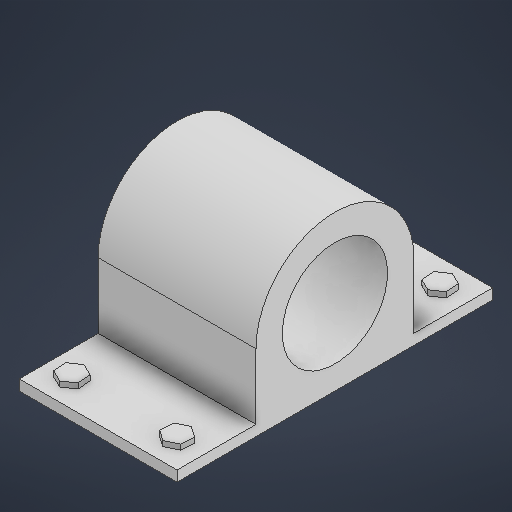
# Autodesk Inventor part: hold down pin
Saved by Autodesk Inventor 2026.1 (Build 301233020, 233B)
## iProperties
Created: 2025-12-30
Part Number: hold down pin
Material: Generic
Document SubType Name: Modeling
Designer: Austin Ngobeni
Density: 1 g/cm^3
Appearance: Default
Author: Austin Ngobeni
Autodesk Inventor part; units mm, degrees
ref_plane "YZ Plane" through (0, 0, 0) normal (1, 0, 0) x (0, 1, 0)
ref_plane "XZ Plane" through (0, 0, 0) normal (0, 1, 0) x (-1, 0, 0)
ref_plane "XY Plane" through (0, 0, 0) normal (0, 0, 1) x (1, 0, 0)
sketch "Sketch1" plane through (0, 0, 0) normal (1, 0, 0) x (0, 1, 0)
  line L0 (-1, 30) -> (1, 30)
  line L1 (1, -30) -> (-1, -30)
  line L2 (-1, -30) -> (-1, 30)
  arc A0 (13.4551, -15) -> (13.4551, 15) centre (13.4551, 0) ccw
  circle A1 centre (13.4551, 0) radius 10
  line L3 (13.4551, 15) -> (1, 15)
  line L4 (13.4551, -15) -> (1, -15)
  line L5 (1, 30) -> (1, 15)
  line L6 (1, -15) -> (1, -30)
  point P0 (0, 0)
  point P1 (0, 30)
  point P2 (1, 0)
  dimension "d0" = 2
  dimension "d1" = 60
  dimension "d2" = 30
  dimension "d3" = 20
  constraints: 14 end point, 4 perpendicular, 3 parallel, 2 centre point, 2 horizontal, 2 point on circle, 2 tangent, 1 coincident, 1 horizontal alignment, 1 midpoint, 1 vertical alignment
  measures "d0" distance of L0.start L0.end
  measures "d1" distance of L0.end L1.start
  measures "d2" diameter of A0
  measures "d3" diameter of A1
extrude "Extrusion1" add sketch "Sketch1" along normal blind 30
sketch "Sketch2" plane through (0, 1, 30) normal (0, 1, 0) x (1, 0, 0)
  circle A0 centre (5, 5) radius 2.5 construction
  line L0 (0, 0) -> (30, 0) projected
  line L1 (15, 0) -> (15, 91.9575) construction
  line L2 (56.6517, 30) -> (-26.6517, 30) construction
  line L3 (0, 0) -> (0, 60) projected
  line L4 (7.0666, 6.4068) -> (7.2516, 3.9137)
  line L5 (7.2516, 3.9137) -> (5.185, 2.5069)
  line L6 (5.185, 2.5069) -> (2.9334, 3.5932)
  line L7 (2.9334, 3.5932) -> (2.7484, 6.0863)
  line L8 (2.7484, 6.0863) -> (4.815, 7.4931)
  line L9 (4.815, 7.4931) -> (7.0666, 6.4068)
  line L10 (22.9334, 6.4068) -> (22.7484, 3.9137)
  line L11 (22.7484, 3.9137) -> (24.815, 2.5069)
  line L12 (24.815, 2.5069) -> (27.0666, 3.5932)
  line L13 (27.0666, 3.5932) -> (27.2516, 6.0863)
  line L14 (27.2516, 6.0863) -> (25.185, 7.4931)
  line L15 (25.185, 7.4931) -> (22.9334, 6.4068)
  line L16 (7.0666, 53.5932) -> (7.2516, 56.0863)
  line L17 (7.2516, 56.0863) -> (5.185, 57.4931)
  line L18 (5.185, 57.4931) -> (2.9334, 56.4068)
  line L19 (2.9334, 56.4068) -> (2.7484, 53.9137)
  line L20 (2.7484, 53.9137) -> (4.815, 52.5069)
  line L21 (4.815, 52.5069) -> (7.0666, 53.5932)
  line L22 (22.7484, 56.0863) -> (24.815, 57.4931)
  line L23 (22.9334, 53.5932) -> (22.7484, 56.0863)
  line L24 (25.185, 52.5069) -> (22.9334, 53.5932)
  line L25 (27.2516, 53.9137) -> (25.185, 52.5069)
  line L26 (27.0666, 56.4068) -> (27.2516, 53.9137)
  line L27 (24.815, 57.4931) -> (27.0666, 56.4068)
  point P0 (0, 30)
  point P1 (15, 30)
  dimension "d6" = 5
  dimension "d7" = 5
  dimension "d8" = 5
  constraints: 52 end point, 18 symmetric about line, 2 midpoint, 1 coincident, 1 horizontal, 1 point on line, 1 vertical, 16 other
  measures "d7" distance from line of L0 point (5, 5)
  measures "d8" distance from line of L3 point (5, 5)
extrude "Extrusion2" add sketch "Sketch2" along normal blind 1
body "Solid1"
